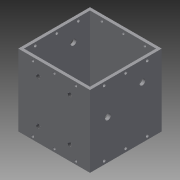
# Autodesk Inventor part: Left_Parallel_Case
Saved by Autodesk Inventor 2013 (Build 170138000, 138)
## iProperties
Created: 2014-02-01
Material: 一般
Document SubType Name: Modeling
Designer: andou
Density: 1 g/cm^3
Mass: 16.8573 g
Surface Area: 190.608 cm^2
Volume: 16.8573 cm^3
Author: andou
Title: Left_Parallel_Case
Autodesk Inventor part; units mm, degrees
ref_plane "YZ Plane" through (0, 0, 0) normal (1, 0, 0) x (0, 1, 0)
ref_plane "XZ Plane" through (0, 0, 0) normal (0, 1, 0) x (-1, 0, 0)
ref_plane "XY Plane" through (0, 0, 0) normal (0, 0, 1) x (1, 0, 0)
sketch "スケッチ1" plane through (0, 0, 0) normal (0, 0, 1) x (1, 0, 0)
  line L0 (-25, 25) -> (25, 25)
  line L1 (25, 25) -> (25, -25)
  line L2 (25, -25) -> (-25, -25)
  line L3 (-25, -25) -> (-25, 25)
  line L4 (-23, 23) -> (23, 23)
  line L5 (23, 23) -> (23, -23)
  line L6 (23, -23) -> (-23, -23)
  line L7 (-23, -23) -> (-23, 23)
  point P0 (0, 0)
  dimension "d0" = 50
  dimension "d1" = 50
  dimension "d4" = 25
  dimension "d5" = 25
  dimension "d6" = 46
  dimension "d7" = 2
  dimension "d8" = 46
  dimension "d9" = 2
  constraints: 16 end point, 4 parallel, 2 horizontal, 2 perpendicular
  measures "d0" distance of L0.start L0.end
  measures "d1" distance of L2.end L0.start
  measures "d4" distance from line of L0 point (0, 0)
  measures "d5" distance from line of L3 point (0, 0)
  measures "d6" distance between parallel lines of L5 L7
  measures "d7" distance between parallel lines of L3 L7
  measures "d8" distance between parallel lines of L4 L6
  measures "d9" distance between parallel lines of L2 L6
extrude "押し出し1" add sketch "スケッチ1" along normal blind 50
sketch "スケッチ11" plane through (25, -25, 0) normal (1, 0, 0) x (0, 0, -1)
  circle A0 centre (-36.5, 36.5) radius 1.5
  line L0 (-50, 50) -> (-50, 0) projected
  circle A1 centre (-27.5, 12.5) radius 1.5
  line L1 (0, 50) -> (0, 0) projected
  line L2 (0, 50) -> (-50, 50) projected
  point P0 (0, 25)
  point P1 (-50, 43)
  dimension "d192" = 118
  dimension "d109" = 3
  dimension "d128" = 24
  dimension "d237" = 13.5
  dimension "d238" = 27.5
  dimension "d239" = 13.5
  constraints: 2 centre point, 1 equal radius
  measures "d109" diameter of A0
  measures "d128" vertical distance of A1.centre A0.centre
  measures "d237" distance from line of L2 A0.centre
  measures "d238" distance from line of L1 A1.centre
  measures "d239" distance from line of L0 A0.centre
hole "穴6" at (25, -12.5, 27.5) at (25, 11.5, 36.5) direction (-1, 0, 0) diameter 4 end through all
sketch "スケッチ15" plane through (-25, -25, 0) normal (0, -1, 0) x (1, 0, 0)
  line L0 (50, 50) -> (0, 50) projected
  line L1 (0, 0) -> (0, 50) projected
  circle A0 centre (10, 47.75) radius 1
  circle A1 centre (25, 47.75) radius 1
  circle A2 centre (40, 47.75) radius 1
  line L2 (50, 0) -> (0, 0) projected
  circle A3 centre (10, 2.25) radius 1
  circle A4 centre (25, 2.25) radius 1
  circle A5 centre (40, 2.25) radius 1
  point P0 (49.5, 0)
  point P1 (49.5, 50)
  point P2 (25, 0)
  dimension "d138" = 2
  dimension "d139" = 10
  dimension "d141" = 2.25
  dimension "d142" = 2.25
  dimension "d143" = 2.25
  dimension "d144" = 15
  dimension "d166" = 15
  dimension "d167" = 10
  dimension "d168" = 15
  dimension "d169" = 15
  dimension "d170" = 2.25
  dimension "d171" = 2.25
  dimension "d172" = 2.25
  constraints: 6 centre point, 5 equal radius
  measures "d138" diameter of A0
  measures "d139" distance from line of L1 A0.centre
  measures "d141" distance from line of L0 A0.centre
  measures "d142" distance from line of L0 A1.centre
  measures "d143" distance from line of L0 A2.centre
  measures "d144" distance of A0.centre A1.centre
  measures "d166" distance of A4.centre A3.centre
  measures "d167" distance from line of L1 A3.centre
  measures "d168" distance of A4.centre A5.centre
  measures "d169" distance of A1.centre A2.centre
  measures "d170" distance from line of L2 A3.centre
  measures "d171" distance from line of A4.centre L2
  measures "d172" distance from line of A5.centre L2
hole "穴10" at (-15, -25, 47.75) at (-15, -25, 2.25) at (0, -25, 47.75) at (0, -25, 2.25) at (15, -25, 2.25) at (15, -25, 47.75) direction (0, 1, 0) diameter 2 end through all
sketch "スケッチ16" plane through (-25, -25, 0) normal (-1, 0, 0) x (0, 0, 1)
  line L0 (50, 0) -> (50, 50) projected
  line L1 (0, 50) -> (50, 50) projected
  line L2 (0, 0) -> (50, 0) projected
  circle A0 centre (47.75, 40) radius 1
  circle A1 centre (47.75, 25) radius 1
  circle A2 centre (47.75, 10) radius 1
  circle A3 centre (2.25, 40) radius 1
  circle A4 centre (2.25, 25) radius 1
  circle A5 centre (2.25, 10) radius 1
  line L3 (0, 48) -> (0, 2) projected
  point P0 (0, 25)
  dimension "d152" = 2
  dimension "d153" = 2.25
  dimension "d154" = 2.25
  dimension "d155" = 2.25
  dimension "d156" = 10
  dimension "d157" = 10
  dimension "d158" = 15
  dimension "d173" = 15
  dimension "d174" = 15
  dimension "d175" = 10
  dimension "d176" = 2.25
  dimension "d177" = 2.25
  dimension "d178" = 2.25
  constraints: 6 centre point, 5 equal radius
  measures "d152" diameter of A0
  measures "d153" distance from line of L0 A0.centre
  measures "d154" distance from line of L0 A1.centre
  measures "d155" distance from line of L0 A2.centre
  measures "d156" distance from line of L2 A2.centre
  measures "d157" distance from line of L1 A0.centre
  measures "d158" distance of A0.centre A1.centre
  measures "d173" distance of A3.centre A4.centre
  measures "d174" distance of A4.centre A5.centre
  measures "d175" distance from line of L1 A3.centre
  measures "d176" distance from line of L3 A3.centre
  measures "d177" distance from line of L3 A4.centre
  measures "d178" distance from line of L3 A5.centre
hole "穴11" at (-25, 15, 2.25) at (-25, 0, 2.25) at (-25, -15, 2.25) at (-25, -15, 47.75) at (-25, 0, 47.75) at (-25, 15, 47.75) direction (1, 0, 0) diameter 2 end through all
sketch "スケッチ18" plane through (-25, -25, 0) normal (0, -1, 0) x (1, 0, 0)
  circle A0 centre (25, 2.25) radius 1 projected
  circle A1 centre (25, 47.75) radius 1 projected
  line L0 (50, 50) -> (0, 50) projected
  line L1 (50, 0) -> (0, 0) projected
  circle A2 centre (14, 40) radius 1.5
  circle A3 centre (36, 40) radius 1.5
  circle A4 centre (14, 10) radius 1.5
  circle A5 centre (36, 10) radius 1.5
  point P0 (49.5, 0)
  point P1 (49.5, 50)
  point P2 (25, 0)
  dimension "d240" = 10
  dimension "d241" = 10
  dimension "d242" = 10
  dimension "d243" = 10
  dimension "d244" = 11
  dimension "d245" = 11
  dimension "d246" = 11
  dimension "d247" = 11
  dimension "d248" = 3
  constraints: 4 centre point, 3 equal radius
  measures "d240" distance from line of L1 A4.centre
  measures "d241" distance from line of L1 A5.centre
  measures "d242" distance from line of L0 A2.centre
  measures "d243" distance from line of L0 A3.centre
  measures "d244" horizontal distance of A1.centre A3.centre
  measures "d245" horizontal distance of A2.centre A1.centre
  measures "d246" horizontal distance of point (25, 0) A4.centre
  measures "d247" horizontal distance of A0.centre A5.centre
  measures "d248" diameter of A5
hole "穴13" at (-11, -25, 40) at (-11, -25, 10) at (11, -25, 40) at (11, -25, 10) direction (0, 1, 0) diameter 3 depth 2 tip angle 118
thread "ねじ13" size "M3x0.5" class "6H" standard "ANSI Metric M Profile" full length
thread "ねじ14" size "M3x0.5" class "6H" standard "ANSI Metric M Profile" full length
thread "ねじ15" size "M3x0.5" class "6H" standard "ANSI Metric M Profile" full length
thread "ねじ16" size "M3x0.5" class "6H" standard "ANSI Metric M Profile" full length
